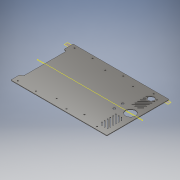
# Autodesk Inventor part: Back
Saved by Autodesk Inventor 2018 (Build 220112000, 112)
## iProperties
Created: 2017-11-12
Part Number: Back
Material: Edelstahl
Document SubType Name: Blech
Density: 8 g/cm^3
Sheet Metal Rule: Standard_mm
Appearance: Halbpoliert
Flat Pattern Width: 22.4 cm
Flat Pattern Length: 34.5 cm
Flat Pattern Area: 772.799 cm^2
Sheet Metal Width: 224,000 mm
Sheet Metal Length: 345,000 mm
Sheet Metal Area: 77279,943 mm^2
Autodesk Inventor part; units mm, degrees
ref_plane "YZ Plane" through (0, 0, 0) normal (1, 0, 0) x (0, 1, 0)
ref_plane "XZ Plane" through (0, 0, 0) normal (0, 1, 0) x (-1, 0, 0)
ref_plane "XY Plane" through (0, 0, 0) normal (0, 0, 1) x (1, 0, 0)
ref_plane "Arbeitsebene1" through (0, 0, 0) normal (0, 0, 1) x (1, 0, 0)
sketch "Skizze1" plane through (0, 0, 0) normal (0, 0, 1) x (1, 0, 0)
  circle A0 centre (70.3399, -192.2557) radius 2.15 construction
  circle A1 centre (-29.6601, -192.2557) radius 2.15 construction
  circle A2 centre (-29.6601, -17.2557) radius 2.15 construction
  circle A3 centre (70.3399, -17.2557) radius 2.15 construction
  arc A4 (-167.6601, 7.2442) -> (-169.6601, 5.2442) centre (-167.6601, 5.2442) ccw construction
  line L0 (-167.6601, 7.2442) -> (173.3399, 7.2442) construction
  arc A5 (175.3399, 5.2442) -> (173.3399, 7.2442) centre (173.3399, 5.2442) ccw construction
  line L1 (175.3399, -214.7557) -> (175.3399, 5.2442) construction
  arc A6 (173.3399, -216.7557) -> (175.3399, -214.7557) centre (173.3399, -214.7557) ccw construction
  line L2 (-167.6601, -216.7557) -> (173.3399, -216.7557) construction
  arc A7 (-169.6601, -214.7557) -> (-167.6601, -216.7557) centre (-167.6601, -214.7557) ccw construction
  line L3 (-169.6601, -188.2557) -> (-169.6601, -214.7557) construction
  arc A8 (-167.6601, -186.2557) -> (-169.6601, -188.2557) centre (-167.6601, -188.2557) ccw construction
  line L4 (105.3399, -186.2557) -> (-167.6601, -186.2557) construction
  arc A9 (105.3399, -186.2557) -> (115.3399, -176.2557) centre (105.3399, -176.2557) ccw construction
  line L5 (115.3399, -33.2557) -> (115.3399, -176.2557) construction
  arc A10 (115.3399, -33.2557) -> (105.3399, -23.2557) centre (105.3399, -33.2557) ccw construction
  line L6 (-167.6601, -23.2557) -> (105.3399, -23.2557) construction
  arc A11 (-169.6601, -21.2557) -> (-167.6601, -23.2557) centre (-167.6601, -21.2557) ccw construction
  line L7 (-169.6601, 5.2442) -> (-169.6601, -21.2557) construction
  line L8 (175.3399, 7.2442) -> (-169.6601, 7.2442)
  line L9 (-169.6601, 7.2442) -> (-169.6601, -216.7557)
  line L10 (-169.6601, -216.7557) -> (175.3399, -216.7557)
  line L11 (175.3399, -216.7557) -> (175.3399, 7.2442)
  circle A12 centre (-29.6601, -17.2557) radius 2.15
  circle A13 centre (-29.6601, -192.2557) radius 2.15
  circle A14 centre (70.3399, -192.2557) radius 2.15
  circle A15 centre (70.3399, -17.2557) radius 2.15
  circle A16 centre (20.3399, -2.7558) radius 2.15
  circle A17 centre (-89.6601, -206.7557) radius 2.15
  circle A18 centre (130.3399, -206.7557) radius 2.15
  circle A19 centre (20.3399, -206.7557) radius 2.15
  circle A20 centre (-89.6601, -2.7558) radius 2.15
  circle A21 centre (130.3399, -2.7558) radius 2.15
  point P0 (0, 0)
  dimension "d0" = 0
  dimension "d1" = 345
  dimension "d2" = 193.4999
  dimension "d3" = 30.4999
  measures "d0" distance between parallel lines of L1 L11
  measures "d1" distance between parallel lines of L1 L9
  measures "d2" distance between parallel lines of L4 L8
  measures "d3" distance between parallel lines of L4 L10
extrude "Grobblech1" add sketch "Skizze1" along normal blind 2 contours L11 L10 L9 L8 | A16 | A17 | A18 | A19 | A20 | A21
fillet "Eckenrundung1" radius 2 4 edges at (-169.6601, -216.7557, 1) (175.3399, -216.7557, 1) (175.3399, 7.2442, 1) (-169.6601, 7.2442, 1)
sketch "Skizze2" plane through (0, 0, 2) normal (0, 0, 1) x (1, 0, 0)
  arc A0 (-167.6601, 7.2442) -> (-169.6601, 5.2442) centre (-167.6601, 5.2442) ccw projected
  line L0 (-169.6601, -214.7557) -> (-169.6601, 5.2442) projected
  arc A1 (-169.6601, -214.7557) -> (-167.6601, -216.7557) centre (-167.6601, -214.7557) ccw projected
  line L1 (173.3399, -216.7557) -> (-167.6601, -216.7557) projected
  arc A2 (173.3399, -216.7557) -> (175.3399, -214.7557) centre (173.3399, -214.7557) ccw projected
  line L2 (175.3399, 5.2442) -> (175.3399, -214.7557) projected
  arc A3 (175.3399, 5.2442) -> (173.3399, 7.2442) centre (173.3399, 5.2442) ccw projected
  line L3 (-167.6601, 7.2442) -> (173.3399, 7.2442) projected
  circle A4 centre (70.3399, -17.2557) radius 2.15 projected
  circle A5 centre (70.3399, -192.2557) radius 2.15 projected
  circle A6 centre (-29.6601, -192.2557) radius 2.15 projected
  circle A7 centre (-29.6601, -17.2557) radius 2.15 projected
  line L4 (-169.6601, -214.7557) -> (-169.6601, 5.2442) projected
  line L5 (-164.6601, -182.7557) -> (-164.6601, -182.7557)
  line L6 (-164.6601, -26.7558) -> (-164.6601, -26.7558)
  line L7 (-159.6601, -31.7558) -> (-159.6601, -177.7557)
  line L8 (-169.6601, -187.7557) -> (-169.6601, -214.7557)
  line L9 (-169.6601, -21.7558) -> (-169.6601, 5.2442)
  arc A8 (-169.6601, -21.7558) -> (-164.6601, -26.7558) centre (-164.6601, -21.7558) ccw
  arc A9 (-159.6601, -31.7558) -> (-164.6601, -26.7558) centre (-164.6601, -31.7558) ccw
  arc A10 (-164.6601, -182.7557) -> (-159.6601, -177.7557) centre (-164.6601, -177.7557) ccw
  arc A11 (-164.6601, -182.7557) -> (-169.6601, -187.7557) centre (-164.6601, -187.7557) ccw
  line L10 (-169.6601, -21.7558) -> (-169.6601, -187.7557)
  point P0 (0, 0)
  point P1 (-169.6601, -182.7557)
  point P2 (-159.6601, -182.7557)
  point P3 (-169.6601, -26.7558)
  point P4 (-159.6601, -26.7558)
  dimension "d6" = 10
  dimension "d7" = 34
  dimension "d8" = 10
  dimension "d9" = 34
  dimension "d10" = 5
  constraints: 12 end point, 10 point on line, 10 tangent, 8 point on circle, 4 centre point, 3 equal radius, 2 collinear, 1 horizontal, 1 perpendicular
  measures "d6" distance of point (-169.66, -182.756) point (-159.66, -182.756)
  measures "d7" distance between parallel lines of L1 L5
  measures "d8" distance of point (-169.66, -26.756) point (-159.66, -26.756)
  measures "d9" distance between parallel lines of L3 L6
  measures "d10" radius of A8
extrude "Extrusion1" cut sketch "Skizze2" against normal through all contours A8 A9 L7 A10 A11 L0
sketch "Skizze3" plane through (0, 0, 2) normal (0, 0, 1) x (1, 0, 0)
  circle A0 centre (148.5119, -104.7557) radius 16.25 projected
  circle A1 centre (148.5119, -104.7557) radius 17.75
  point P0 (0, 0)
  dimension "d27" = 1.5
  constraints: 1 centre point
  measures "d27" radial gap between concentric circles of A0 A1
extrude "Extrusion2" cut sketch "Skizze3" against normal through all contours A0 | A1
sketch "Skizze4" plane through (0, 0, 2) normal (0, 0, 1) x (1, 0, 0)
  line L0 (115.3399, -201.7557) -> (115.3399, -7.7558) construction
  line L1 (244.3399, -104.7557) -> (-238.6601, -104.7557) construction
  circle A0 centre (105.3399, -119.7557) radius 4
  circle A1 centre (105.3399, -89.7557) radius 4
  point P0 (0, 0)
  dimension "d15" = 8
  dimension "d16" = 8
  dimension "d17" = 15
  dimension "d18" = 10
  dimension "d19" = 10
  dimension "d20" = 15
  constraints: 2 centre point, 2 end point, 1 horizontal, 2 other
  measures "d15" diameter of A0
  measures "d16" diameter of A1
  measures "d17" distance from line of L1 A1.centre
  measures "d18" distance from line of L0 A1.centre
  measures "d19" distance from line of L0 A0.centre
  measures "d20" distance from line of L1 A0.centre
extrude "Extrusion3" cut sketch "Skizze4" against normal through all
sketch "Skizze5" plane through (0, 0, 2) normal (0, 0, 1) x (1, 0, 0)
  circle A0 centre (130.3399, -2.7558) radius 2.15 projected
  circle A1 centre (20.3399, -2.7558) radius 2.15 projected
  circle A2 centre (-89.6601, -2.7558) radius 2.15 projected
  circle A3 centre (-89.6601, -206.7557) radius 2.15 projected
  circle A4 centre (20.3399, -206.7557) radius 2.15 projected
  circle A5 centre (130.3399, -206.7557) radius 2.15 projected
  point P0 (0, 0)
extrude "Extrusion4" cut sketch "Skizze5" against normal through all
ref_plane "Arbeitsebene2" through (-167.6601, -104.7557, 0) normal (0, -1, 0) x (1, 0, 0)
sketch "Skizze6" plane through (0, 0, 0) normal (0, 0, -1) x (-1, 0, 0)
  circle A0 centre (154.6601, -2.7558) radius 2.15
  circle A1 centre (154.6601, -206.7557) radius 2.15
  point P0 (0, 0)
  constraints: 2 centre point, 4 other
extrude "Extrusion5" cut sketch "Skizze6" against normal through all
sketch "Skizze7" plane through (0, 0, 0) normal (0, 0, -1) x (-1, 0, 0)
  line L0 (-97.7459, -78.2296) -> (-73.7459, -78.2296) construction
  line L1 (-70.7459, -75.2296) -> (-70.7459, -21.2296) construction
  line L2 (-73.7459, -18.2296) -> (-97.7459, -18.2296) construction
  line L3 (-100.7459, -21.2296) -> (-100.7459, -75.2296) construction
  circle A0 centre (154.6601, -2.7558) radius 2.15 projected
  circle A1 centre (154.6601, -206.7557) radius 2.15 projected
  circle A2 centre (-20.3399, -206.7557) radius 2.15 projected
  circle A3 centre (89.6601, -2.7558) radius 2.15 projected
  circle A4 centre (-130.3399, -2.7558) radius 2.15 projected
  circle A5 centre (-20.3399, -2.7558) radius 2.15 projected
  circle A6 centre (89.6601, -206.7557) radius 2.15 projected
  circle A7 centre (-130.3399, -206.7557) radius 2.15 projected
  circle A8 centre (-105.3399, -119.7557) radius 4 projected
  circle A9 centre (-105.3399, -89.7557) radius 4 projected
  circle A10 centre (-148.5119, -104.7557) radius 17.75 projected
  arc A11 (169.6601, -187.7557) -> (164.6601, -182.7557) centre (164.6601, -187.7557) ccw projected
  arc A12 (159.6601, -177.7557) -> (164.6601, -182.7557) centre (164.6601, -177.7557) ccw projected
  line L4 (159.6601, -177.7557) -> (159.6601, -31.7558) projected
  arc A13 (164.6601, -26.7558) -> (159.6601, -31.7558) centre (164.6601, -31.7558) ccw projected
  arc A14 (164.6601, -26.7558) -> (169.6601, -21.7558) centre (164.6601, -21.7558) ccw projected
  line L5 (169.6601, 5.2442) -> (169.6601, -21.7558) projected
  arc A15 (169.6601, 5.2442) -> (167.6601, 7.2442) centre (167.6601, 5.2442) ccw projected
  line L6 (-173.3399, 7.2442) -> (167.6601, 7.2442) projected
  arc A16 (-173.3399, 7.2442) -> (-175.3399, 5.2442) centre (-173.3399, 5.2442) ccw projected
  line L7 (-175.3399, -214.7557) -> (-175.3399, 5.2442) projected
  arc A17 (-175.3399, -214.7557) -> (-173.3399, -216.7557) centre (-173.3399, -214.7557) ccw projected
  line L8 (167.6601, -216.7557) -> (-173.3399, -216.7557) projected
  arc A18 (167.6601, -216.7557) -> (169.6601, -214.7557) centre (167.6601, -214.7557) ccw projected
  line L9 (169.6601, -187.7557) -> (169.6601, -214.7557) projected
  circle A19 centre (29.6601, -17.2557) radius 2.15 projected
  circle A20 centre (29.6601, -192.2557) radius 2.15 projected
  circle A21 centre (-70.3399, -192.2557) radius 2.15 projected
  circle A22 centre (-70.3399, -17.2557) radius 2.15 projected
  line L10 (-148.5119, -104.7557) -> (-119.1163, -104.7557) construction
  line L11 (-158.66, -131.2539) -> (-120.76, -131.2539) construction
  arc A23 (-156.5439, -143.3701) -> (-154.7761, -145.1378) centre (-155.66, -144.2539) ccw
  arc A24 (-124.7761, -135.1378) -> (-126.5439, -133.3701) centre (-125.66, -134.2539) ccw
  line L12 (-158.66, -131.2539) -> (-122.66, -131.2539) construction
  line L13 (-156.5439, -173.3701) -> (-126.5439, -143.3701)
  line L14 (-155.66, -174.2539) -> (-125.66, -144.2539) construction
  arc A25 (-124.7761, -175.1378) -> (-126.5439, -173.3701) centre (-125.66, -174.2539) ccw
  line L15 (-156.5439, -183.3701) -> (-126.5439, -153.3701)
  line L16 (-155.66, -184.2539) -> (-125.66, -154.2539) construction
  line L17 (-124.7761, -155.1378) -> (-154.7761, -185.1378)
  line L18 (-155.66, -191.2539) -> (-155.66, -137.2539) construction
  line L19 (-125.66, -137.2539) -> (-125.66, -191.2539) construction
  line L20 (-158.66, -197.2539) -> (-158.66, -131.2539) construction
  line L21 (-122.66, -131.2539) -> (-122.66, -197.2539) construction
  arc A26 (-146.5439, -193.3701) -> (-144.7761, -195.1378) centre (-145.66, -194.2539) ccw
  line L22 (-156.5439, -193.3701) -> (-126.5439, -163.3701)
  line L23 (-155.66, -194.2539) -> (-125.66, -164.2539) construction
  line L24 (-124.7761, -165.1378) -> (-154.7761, -195.1378)
  line L25 (-122.66, -197.2539) -> (-158.66, -197.2539) construction
  arc A27 (-156.5439, -163.3701) -> (-154.7761, -165.1378) centre (-155.66, -164.2539) ccw
  line L26 (-146.5439, -193.3701) -> (-126.5439, -173.3701)
  line L27 (-124.7761, -175.1378) -> (-144.7761, -195.1378)
  arc A28 (-156.5439, -153.3701) -> (-154.7761, -155.1378) centre (-155.66, -154.2539) ccw
  line L28 (-124.7761, -185.1378) -> (-134.7761, -195.1378)
  arc A29 (-156.5439, -173.3701) -> (-154.7761, -175.1378) centre (-155.66, -174.2539) ccw
  arc A30 (-124.7761, -185.1378) -> (-126.5439, -183.3701) centre (-125.66, -184.2539) ccw
  arc A31 (-156.5439, -183.3701) -> (-154.7761, -185.1378) centre (-155.66, -184.2539) ccw
  line L29 (-135.66, -194.2539) -> (-125.66, -184.2539) construction
  line L30 (-145.66, -194.2539) -> (-125.66, -174.2539) construction
  arc A32 (-156.5439, -193.3701) -> (-154.7761, -195.1378) centre (-155.66, -194.2539) ccw
  line L31 (-158.66, -197.8539) -> (-120.76, -197.8539) construction
  arc A33 (-124.7761, -145.1378) -> (-126.5439, -143.3701) centre (-125.66, -144.2539) ccw
  arc A34 (-134.7761, -135.1378) -> (-136.5439, -133.3701) centre (-135.66, -134.2539) ccw
  arc A35 (-125.66, -137.2539) -> (-128.66, -134.2539) centre (-128.66, -137.2539) ccw construction
  arc A36 (-144.7761, -135.1378) -> (-146.5439, -133.3701) centre (-145.66, -134.2539) ccw
  arc A37 (-124.7761, -165.1378) -> (-126.5439, -163.3701) centre (-125.66, -164.2539) ccw
  line L32 (-152.66, -134.2539) -> (-128.66, -134.2539) construction
  arc A38 (-152.66, -134.2539) -> (-155.66, -137.2539) centre (-152.66, -137.2539) ccw construction
  line L33 (-144.7761, -135.1378) -> (-154.7761, -145.1378)
  line L34 (-155.66, -144.2539) -> (-145.66, -134.2539) construction
  line L35 (-156.5439, -143.3701) -> (-146.5439, -133.3701)
  line L36 (-134.7761, -135.1378) -> (-154.7761, -155.1378)
  line L37 (-155.66, -154.2539) -> (-135.66, -134.2539) construction
  line L38 (-156.5439, -153.3701) -> (-136.5439, -133.3701)
  line L39 (-156.5439, -163.3701) -> (-126.5439, -133.3701)
  line L40 (-155.66, -164.2539) -> (-125.66, -134.2539) construction
  line L41 (-124.7761, -135.1378) -> (-154.7761, -165.1378)
  line L42 (-124.7761, -145.1378) -> (-154.7761, -175.1378)
  arc A39 (-124.7761, -155.1378) -> (-126.5439, -153.3701) centre (-125.66, -154.2539) ccw
  line L43 (-128.66, -194.2539) -> (-152.66, -194.2539) construction
  arc A40 (-128.66, -194.2539) -> (-125.66, -191.2539) centre (-128.66, -191.2539) ccw construction
  line L44 (-136.5439, -193.3701) -> (-126.5439, -183.3701)
  arc A41 (-155.66, -191.2539) -> (-152.66, -194.2539) centre (-152.66, -191.2539) ccw construction
  arc A42 (-136.5439, -193.3701) -> (-134.7761, -195.1378) centre (-135.66, -194.2539) ccw
  line L45 (-175.3399, -214.7557) -> (-175.3399, 5.2442) projected
  line L46 (-173.3399, -203.5364) -> (-171.4999, -203.5364) construction
  arc A43 (-154.7761, -34.3737) -> (-156.5439, -36.1414) centre (-155.66, -35.2576) ccw
  arc A44 (-154.7761, -44.3737) -> (-156.5439, -46.1414) centre (-155.66, -45.2576) ccw
  arc A45 (-155.66, -72.2576) -> (-152.66, -75.2576) centre (-152.66, -72.2576) ccw construction
  line L47 (-155.66, -65.2576) -> (-145.66, -75.2576) construction
  line L48 (-156.5439, -16.1414) -> (-126.5439, -46.1414)
  arc A46 (-128.66, -75.2576) -> (-125.66, -72.2576) centre (-128.66, -72.2576) ccw construction
  arc A47 (-136.5439, -76.1414) -> (-134.7761, -74.3737) centre (-135.66, -75.2576) ccw
  arc A48 (-154.7761, -54.3737) -> (-156.5439, -56.1414) centre (-155.66, -55.2576) ccw
  line L49 (-158.66, -12.2576) -> (-158.66, -78.2576) construction
  line L50 (-124.7761, -34.3737) -> (-144.7761, -14.3737)
  line L51 (-122.66, -12.2576) -> (-158.66, -12.2576) construction
  arc A49 (-126.5439, -26.1414) -> (-124.7761, -24.3737) centre (-125.66, -25.2576) ccw
  arc A50 (-126.5439, -66.1414) -> (-124.7761, -64.3737) centre (-125.66, -65.2576) ccw
  line L52 (-122.66, -78.2576) -> (-122.66, -12.2576) construction
  arc A51 (-126.5439, -36.1414) -> (-124.7761, -34.3737) centre (-125.66, -35.2576) ccw
  line L53 (-158.66, -78.2576) -> (-120.76, -78.2576) construction
  line L54 (-156.5439, -36.1414) -> (-126.5439, -66.1414)
  arc A52 (-154.7761, -64.3737) -> (-156.5439, -66.1414) centre (-155.66, -65.2576) ccw
  arc A53 (-126.5439, -76.1414) -> (-124.7761, -74.3737) centre (-125.66, -75.2576) ccw
  line L55 (-158.66, -78.2576) -> (-122.66, -78.2576) construction
  arc A54 (-126.5439, -46.1414) -> (-124.7761, -44.3737) centre (-125.66, -45.2576) ccw
  arc A55 (-146.5439, -76.1414) -> (-144.7761, -74.3737) centre (-145.66, -75.2576) ccw
  arc A56 (-125.66, -18.2576) -> (-128.66, -15.2576) centre (-128.66, -18.2576) ccw construction
  line L56 (-124.7761, -44.3737) -> (-154.7761, -14.3737)
  line L57 (-158.66, -11.6576) -> (-120.76, -11.6576) construction
  line L58 (-124.7761, -24.3737) -> (-134.7761, -14.3737)
  line L59 (-144.7761, -74.3737) -> (-154.7761, -64.3737)
  line L60 (-152.66, -75.2576) -> (-128.66, -75.2576) construction
  arc A57 (-134.7761, -14.3737) -> (-136.5439, -16.1414) centre (-135.66, -15.2576) ccw
  line L61 (-136.5439, -16.1414) -> (-126.5439, -26.1414)
  line L62 (-135.66, -15.2576) -> (-125.66, -25.2576) construction
  line L63 (-145.66, -15.2576) -> (-125.66, -35.2576) construction
  arc A58 (-144.7761, -14.3737) -> (-146.5439, -16.1414) centre (-145.66, -15.2576) ccw
  line L64 (-128.66, -15.2576) -> (-152.66, -15.2576) construction
  arc A59 (-152.66, -15.2576) -> (-155.66, -18.2576) centre (-152.66, -18.2576) ccw construction
  arc A60 (-126.5439, -56.1414) -> (-124.7761, -54.3737) centre (-125.66, -55.2576) ccw
  line L65 (-124.7761, -54.3737) -> (-154.7761, -24.3737)
  line L66 (-155.66, -25.2576) -> (-125.66, -55.2576) construction
  line L67 (-156.5439, -26.1414) -> (-126.5439, -56.1414)
  line L68 (-125.66, -72.2576) -> (-125.66, -18.2576) construction
  line L69 (-155.66, -18.2576) -> (-155.66, -72.2576) construction
  line L70 (-124.7761, -64.3737) -> (-154.7761, -34.3737)
  line L71 (-155.66, -35.2576) -> (-125.66, -65.2576) construction
  line L72 (-124.7761, -74.3737) -> (-154.7761, -44.3737)
  line L73 (-155.66, -45.2576) -> (-125.66, -75.2576) construction
  line L74 (-156.5439, -46.1414) -> (-126.5439, -76.1414)
  line L75 (-134.7761, -74.3737) -> (-154.7761, -54.3737)
  line L76 (-155.66, -55.2576) -> (-135.66, -75.2576) construction
  line L77 (-156.5439, -56.1414) -> (-136.5439, -76.1414)
  line L78 (-156.5439, -66.1414) -> (-146.5439, -76.1414)
  line L79 (-146.5439, -16.1414) -> (-126.5439, -36.1414)
  line L80 (-155.66, -15.2576) -> (-125.66, -45.2576) construction
  arc A61 (-154.7761, -14.3737) -> (-156.5439, -16.1414) centre (-155.66, -15.2576) ccw
  arc A62 (-154.7761, -24.3737) -> (-156.5439, -26.1414) centre (-155.66, -25.2576) ccw
  point P0 (0, 0)
  point P1 (-100.7459, -78.2296)
  point P2 (-100.7459, -68.2296)
  point P3 (-100.7459, -58.2296)
  point P4 (-100.7459, -48.2296)
  point P5 (-100.7459, -38.2296)
  point P6 (-100.7459, -28.2296)
  point P7 (-100.7459, -18.2296)
  point P8 (-90.7459, -78.2296)
  point P9 (-80.7459, -78.2296)
  point P10 (-70.7459, -78.2296)
  point P11 (-70.7459, -68.2296)
  point P12 (-70.7459, -58.2296)
  point P13 (-70.7459, -48.2296)
  point P14 (-70.7459, -38.2296)
  point P15 (-70.7459, -28.2296)
  point P16 (-70.7459, -18.2296)
  point P17 (-90.7459, -18.2296)
  point P18 (-80.7459, -18.2296)
  point P19 (-70.7459, -18.2296)
  point P20 (-155.66, -134.2539)
  point P21 (-125.66, -134.2539)
  point P22 (-140.66, -179.2539)
  point P23 (-140.66, -149.2539)
  point P24 (-145.66, -144.2539)
  point P25 (-150.66, -139.2539)
  point P26 (-140.66, -169.2539)
  point P27 (-140.66, -159.2539)
  point P28 (-135.66, -184.2539)
  point P29 (-130.66, -189.2539)
  point P30 (-125.66, -194.2539)
  point P31 (-135.66, -194.2539)
  point P32 (-145.66, -194.2539)
  point P33 (-125.66, -194.2539)
  point P34 (-125.66, -184.2539)
  point P35 (-125.66, -174.2539)
  point P36 (-125.66, -164.2539)
  point P37 (-125.66, -154.2539)
  point P38 (-125.66, -144.2539)
  point P39 (-125.66, -134.2539)
  point P40 (-135.66, -134.2539)
  point P41 (-145.66, -134.2539)
  point P42 (-155.66, -194.2539)
  point P43 (-155.66, -184.2539)
  point P44 (-155.66, -174.2539)
  point P45 (-155.66, -164.2539)
  point P46 (-155.66, -154.2539)
  point P47 (-155.66, -144.2539)
  point P48 (-155.66, -134.2539)
  point P49 (-125.66, -75.2576)
  point P50 (-140.66, -60.2576)
  point P51 (-130.66, -20.2576)
  point P52 (-140.66, -50.2576)
  point P53 (-150.66, -70.2576)
  point P54 (-145.66, -65.2576)
  point P55 (-135.66, -25.2576)
  point P56 (-140.66, -40.2576)
  point P57 (-155.66, -75.2576)
  point P58 (-140.66, -30.2576)
  point P59 (-155.66, -75.2576)
  point P60 (-155.66, -65.2576)
  point P61 (-155.66, -55.2576)
  point P62 (-155.66, -45.2576)
  point P63 (-155.66, -35.2576)
  point P64 (-155.66, -25.2576)
  point P65 (-155.66, -15.2576)
  point P66 (-145.66, -75.2576)
  point P67 (-135.66, -75.2576)
  point P68 (-125.66, -75.2576)
  point P69 (-125.66, -65.2576)
  point P70 (-125.66, -55.2576)
  point P71 (-125.66, -45.2576)
  point P72 (-125.66, -35.2576)
  point P73 (-125.66, -25.2576)
  point P74 (-125.66, -15.2576)
  point P75 (-145.66, -15.2576)
  point P76 (-135.66, -15.2576)
  point P77 (-125.66, -15.2576)
  dimension "d50" = 10
  dimension "d51" = 10
  dimension "d52" = 10
  dimension "d53" = 10
  dimension "d71" = 1.84
  constraints: 180 end point, 98 symmetric about line, 80 point on circle, 40 centre point, 12 point on line, 2 horizontal, 2 vertical, 38 other
  measures "d50" distance of point (-100.746, -78.23) point (-100.746, -68.23)
  measures "d51" distance of point (-100.746, -78.23) point (-90.746, -78.23)
  measures "d52" distance of point (-70.746, -78.23) point (-70.746, -68.23)
  measures "d53" distance of point (-100.746, -18.23) point (-90.746, -18.23)
  measures "d71" distance of L46.start L46.end
extrude "Extrusion7" cut sketch "Skizze7" against normal blind 10 contours L35 A36 L33 A23 | L41 A27 L39 A24 | L13 A33 L42 A29 | L27 A26 L26 A25 | L15 A39 L17 A31 | L22 A37 L24 A32 | L38 A34 L36 A28 | L28 A42 L44 A30 | L70 A50 L54 A43 | L72 A53 L74 A44 | A61 L56 A54 L48 | L77 A48 L75 A47 | A51 L79 A58 L50 | L61 A57 L58 A49 | L59 A55 L78 A52 | L67 A62 L65 A60
sketch "Skizze8" plane through (0, 0, 2) normal (0, 0, 1) x (1, 0, 0)
  arc A0 (124.7761, -64.3737) -> (126.5439, -66.1414) centre (125.66, -65.2576) ccw construction
  line L0 (124.7761, -64.3737) -> (154.7761, -34.3737) construction
  arc A1 (156.5439, -36.1414) -> (154.7761, -34.3737) centre (155.66, -35.2576) ccw construction
  line L1 (156.5439, -36.1414) -> (126.5439, -66.1414) construction
  arc A2 (124.7761, -74.3737) -> (126.5439, -76.1414) centre (125.66, -75.2576) ccw construction
  line L2 (124.7761, -74.3737) -> (154.7761, -44.3737) construction
  arc A3 (156.5439, -46.1414) -> (154.7761, -44.3737) centre (155.66, -45.2576) ccw construction
  line L3 (156.5439, -46.1414) -> (126.5439, -76.1414) construction
  arc A4 (126.5439, -133.3701) -> (124.7761, -135.1378) centre (125.66, -134.2539) ccw projected
  line L4 (126.5439, -133.3701) -> (156.5439, -163.3701) projected
  arc A5 (154.7761, -165.1378) -> (156.5439, -163.3701) centre (155.66, -164.2539) ccw projected
  line L5 (154.7761, -165.1378) -> (124.7761, -135.1378) projected
  arc A6 (126.5439, -153.3701) -> (124.7761, -155.1378) centre (125.66, -154.2539) ccw projected
  line L6 (126.5439, -153.3701) -> (156.5439, -183.3701) projected
  arc A7 (154.7761, -185.1378) -> (156.5439, -183.3701) centre (155.66, -184.2539) ccw projected
  line L7 (154.7761, -185.1378) -> (124.7761, -155.1378) projected
  arc A8 (146.5439, -16.1414) -> (144.7761, -14.3737) centre (145.66, -15.2576) ccw construction
  line L8 (146.5439, -16.1414) -> (126.5439, -36.1414) construction
  arc A9 (124.7761, -34.3737) -> (126.5439, -36.1414) centre (125.66, -35.2576) ccw construction
  line L9 (124.7761, -34.3737) -> (144.7761, -14.3737) construction
  arc A10 (136.5439, -133.3701) -> (134.7761, -135.1378) centre (135.66, -134.2539) ccw projected
  line L10 (136.5439, -133.3701) -> (156.5439, -153.3701) projected
  arc A11 (154.7761, -155.1378) -> (156.5439, -153.3701) centre (155.66, -154.2539) ccw projected
  line L11 (154.7761, -155.1378) -> (134.7761, -135.1378) projected
  arc A12 (124.7761, -24.3737) -> (126.5439, -26.1414) centre (125.66, -25.2576) ccw construction
  line L12 (124.7761, -24.3737) -> (134.7761, -14.3737) construction
  arc A13 (136.5439, -16.1414) -> (134.7761, -14.3737) centre (135.66, -15.2576) ccw construction
  line L13 (136.5439, -16.1414) -> (126.5439, -26.1414) construction
  arc A14 (134.7761, -195.1378) -> (136.5439, -193.3701) centre (135.66, -194.2539) ccw projected
  line L14 (134.7761, -195.1378) -> (124.7761, -185.1378) projected
  arc A15 (126.5439, -183.3701) -> (124.7761, -185.1378) centre (125.66, -184.2539) ccw projected
  line L15 (126.5439, -183.3701) -> (136.5439, -193.3701) projected
  arc A16 (146.5439, -133.3701) -> (144.7761, -135.1378) centre (145.66, -134.2539) ccw projected
  line L16 (146.5439, -133.3701) -> (156.5439, -143.3701) projected
  arc A17 (154.7761, -145.1378) -> (156.5439, -143.3701) centre (155.66, -144.2539) ccw projected
  line L17 (154.7761, -145.1378) -> (144.7761, -135.1378) projected
  arc A18 (156.5439, -66.1414) -> (154.7761, -64.3737) centre (155.66, -65.2576) ccw construction
  line L18 (156.5439, -66.1414) -> (146.5439, -76.1414) construction
  arc A19 (144.7761, -74.3737) -> (146.5439, -76.1414) centre (145.66, -75.2576) ccw construction
  line L19 (144.7761, -74.3737) -> (154.7761, -64.3737) construction
  arc A20 (126.5439, -173.3701) -> (124.7761, -175.1378) centre (125.66, -174.2539) ccw projected
  line L20 (126.5439, -173.3701) -> (146.5439, -193.3701) projected
  arc A21 (144.7761, -195.1378) -> (146.5439, -193.3701) centre (145.66, -194.2539) ccw projected
  line L21 (144.7761, -195.1378) -> (124.7761, -175.1378) projected
  arc A22 (156.5439, -56.1414) -> (154.7761, -54.3737) centre (155.66, -55.2576) ccw construction
  line L22 (156.5439, -56.1414) -> (136.5439, -76.1414) construction
  arc A23 (134.7761, -74.3737) -> (136.5439, -76.1414) centre (135.66, -75.2576) ccw construction
  line L23 (134.7761, -74.3737) -> (154.7761, -54.3737) construction
  arc A24 (154.7761, -195.1378) -> (156.5439, -193.3701) centre (155.66, -194.2539) ccw projected
  line L24 (154.7761, -195.1378) -> (124.7761, -165.1378) projected
  arc A25 (126.5439, -163.3701) -> (124.7761, -165.1378) centre (125.66, -164.2539) ccw projected
  line L25 (126.5439, -163.3701) -> (156.5439, -193.3701) projected
  arc A26 (126.5439, -143.3701) -> (124.7761, -145.1378) centre (125.66, -144.2539) ccw projected
  line L26 (126.5439, -143.3701) -> (156.5439, -173.3701) projected
  arc A27 (154.7761, -175.1378) -> (156.5439, -173.3701) centre (155.66, -174.2539) ccw projected
  line L27 (154.7761, -175.1378) -> (124.7761, -145.1378) projected
  arc A28 (156.5439, -26.1414) -> (154.7761, -24.3737) centre (155.66, -25.2576) ccw construction
  line L28 (156.5439, -26.1414) -> (126.5439, -56.1414) construction
  arc A29 (124.7761, -54.3737) -> (126.5439, -56.1414) centre (125.66, -55.2576) ccw construction
  line L29 (124.7761, -54.3737) -> (154.7761, -24.3737) construction
  arc A30 (124.7761, -44.3737) -> (126.5439, -46.1414) centre (125.66, -45.2576) ccw construction
  line L30 (124.7761, -44.3737) -> (154.7761, -14.3737) construction
  arc A31 (156.5439, -16.1414) -> (154.7761, -14.3737) centre (155.66, -15.2576) ccw construction
  line L31 (156.5439, -16.1414) -> (126.5439, -46.1414) construction
  circle A32 centre (-154.6601, -2.7558) radius 2.15 projected
  circle A33 centre (-154.6601, -206.7557) radius 2.15 projected
  circle A34 centre (20.3399, -206.7557) radius 2.15 projected
  circle A35 centre (-89.6601, -2.7558) radius 2.15 projected
  circle A36 centre (130.3399, -2.7558) radius 2.15 projected
  circle A37 centre (20.3399, -2.7558) radius 2.15 projected
  circle A38 centre (-89.6601, -206.7557) radius 2.15 projected
  circle A39 centre (130.3399, -206.7557) radius 2.15 projected
  circle A40 centre (105.3399, -119.7557) radius 4 projected
  circle A41 centre (105.3399, -89.7557) radius 4 projected
  circle A42 centre (148.5119, -104.7557) radius 17.75 projected
  arc A43 (-164.6601, -182.7557) -> (-169.6601, -187.7557) centre (-164.6601, -187.7557) ccw projected
  line L32 (-169.6601, -214.7557) -> (-169.6601, -187.7557) projected
  arc A44 (-169.6601, -214.7557) -> (-167.6601, -216.7557) centre (-167.6601, -214.7557) ccw projected
  line L33 (173.3399, -216.7557) -> (-167.6601, -216.7557) projected
  arc A45 (173.3399, -216.7557) -> (175.3399, -214.7557) centre (173.3399, -214.7557) ccw projected
  line L34 (175.3399, 5.2442) -> (175.3399, -214.7557) projected
  arc A46 (175.3399, 5.2442) -> (173.3399, 7.2442) centre (173.3399, 5.2442) ccw projected
  line L35 (-167.6601, 7.2442) -> (173.3399, 7.2442) projected
  arc A47 (-167.6601, 7.2442) -> (-169.6601, 5.2442) centre (-167.6601, 5.2442) ccw projected
  line L36 (-169.6601, -21.7558) -> (-169.6601, 5.2442) projected
  arc A48 (-169.6601, -21.7558) -> (-164.6601, -26.7558) centre (-164.6601, -21.7558) ccw projected
  arc A49 (-159.6601, -31.7558) -> (-164.6601, -26.7558) centre (-164.6601, -31.7558) ccw projected
  line L37 (-159.6601, -31.7558) -> (-159.6601, -177.7557) projected
  arc A50 (-164.6601, -182.7557) -> (-159.6601, -177.7557) centre (-164.6601, -177.7557) ccw projected
  circle A51 centre (70.3399, -17.2557) radius 2.15 projected
  circle A52 centre (70.3399, -192.2557) radius 2.15 projected
  circle A53 centre (-29.6601, -192.2557) radius 2.15 projected
  circle A54 centre (-29.6601, -17.2557) radius 2.15 projected
  line L38 (155.66, -15.2576) -> (125.66, -15.2576) construction
  line L39 (125.66, -15.2576) -> (125.66, -75.2576) construction
  line L40 (125.66, -75.2576) -> (155.66, -75.2576) construction
  line L41 (155.66, -75.2576) -> (155.66, -15.2576) construction
  line L42 (155.66, -15.2576) -> (125.66, -75.2576) construction
  line L43 (125.66, -15.2576) -> (155.66, -75.2576) construction
  circle A55 centre (140.66, -22.7558) radius 13.75
  circle A56 centre (130.3399, -2.7558) radius 3.75 construction
  point P0 (0, 0)
  dimension "d75" = 27.5
  dimension "d76" = 34.6799
  dimension "d77" = 30
  dimension "d83" = 7.5
  constraints: 12 end point, 2 centre point, 2 parallel, 1 coincident, 1 horizontal, 1 perpendicular
  measures "d75" diameter of A55
  measures "d76" distance from line of L34 A55.centre
  measures "d77" distance from line of L35 A55.centre
  measures "d83" diameter of A56
extrude "Extrusion8" add sketch "Skizze8" against normal blind 2 contours A55
sketch "Skizze9" plane through (0, 0, 2) normal (0, 0, 1) x (1, 0, 0)
  line L0 (156.5439, -46.1414) -> (126.5439, -76.1414) projected
  arc A0 (124.7761, -74.3737) -> (126.5439, -76.1414) centre (125.66, -75.2576) ccw projected
  line L1 (124.7761, -74.3737) -> (154.7761, -44.3737) projected
  arc A1 (126.9201, -22.2297) -> (127.1864, -25.4989) centre (140.66, -22.7558) ccw construction
  line L2 (156.5439, -36.1414) -> (126.5439, -66.1414) projected
  arc A2 (124.7761, -64.3737) -> (126.5439, -66.1414) centre (125.66, -65.2576) ccw projected
  line L3 (124.7761, -64.3737) -> (154.7761, -34.3737) projected
  arc A3 (129.0411, -30.1087) -> (130.5789, -32.1064) centre (140.66, -22.7558) ccw projected
  line L4 (148.9898, -33.6955) -> (126.5439, -56.1414) projected
  arc A4 (124.7761, -54.3737) -> (126.5439, -56.1414) centre (125.66, -55.2576) ccw projected
  line L5 (124.7761, -54.3737) -> (142.8137, -36.3361) projected
  arc A5 (142.8137, -36.3361) -> (148.9898, -33.6955) centre (140.66, -22.7558) ccw projected
  line L6 (136.7478, -35.9375) -> (126.5439, -46.1414) projected
  arc A6 (124.7761, -44.3737) -> (126.5439, -46.1414) centre (125.66, -45.2576) ccw projected
  line L7 (124.7761, -44.3737) -> (134.2366, -34.9132) projected
  arc A7 (134.2366, -34.9132) -> (136.7478, -35.9375) centre (140.66, -22.7558) ccw projected
  arc A8 (156.5439, -46.1414) -> (154.7761, -44.3737) centre (155.66, -45.2576) ccw projected
  arc A9 (156.5439, -36.1414) -> (154.7761, -34.3737) centre (155.66, -35.2576) ccw projected
  arc A10 (151.5997, -31.0856) -> (154.2403, -24.9095) centre (140.66, -22.7558) ccw projected
  line L8 (154.2403, -24.9095) -> (154.7761, -24.3737) projected
  arc A11 (156.5439, -26.1414) -> (154.7761, -24.3737) centre (155.66, -25.2576) ccw projected
  line L9 (156.5439, -26.1414) -> (151.5997, -31.0856) projected
  arc A12 (153.8417, -18.8436) -> (152.8174, -16.3324) centre (140.66, -22.7558) ccw projected
  line L10 (152.8174, -16.3324) -> (154.7761, -14.3737) projected
  arc A13 (156.5439, -16.1414) -> (154.7761, -14.3737) centre (155.66, -15.2576) ccw projected
  line L11 (156.5439, -16.1414) -> (153.8417, -18.8436) projected
  arc A14 (126.5439, -133.3701) -> (124.7761, -135.1378) centre (125.66, -134.2539) ccw projected
  line L12 (126.5439, -133.3701) -> (156.5439, -163.3701) projected
  arc A15 (154.7761, -165.1378) -> (156.5439, -163.3701) centre (155.66, -164.2539) ccw projected
  line L13 (154.7761, -165.1378) -> (124.7761, -135.1378) projected
  arc A16 (126.5439, -153.3701) -> (124.7761, -155.1378) centre (125.66, -154.2539) ccw projected
  line L14 (126.5439, -153.3701) -> (156.5439, -183.3701) projected
  arc A17 (154.7761, -185.1378) -> (156.5439, -183.3701) centre (155.66, -184.2539) ccw projected
  line L15 (154.7761, -185.1378) -> (124.7761, -155.1378) projected
  line L16 (130.5789, -32.1064) -> (126.5439, -36.1414) projected
  arc A18 (124.7761, -34.3737) -> (126.5439, -36.1414) centre (125.66, -35.2576) ccw projected
  line L17 (124.7761, -34.3737) -> (129.0411, -30.1087) projected
  arc A19 (136.5439, -133.3701) -> (134.7761, -135.1378) centre (135.66, -134.2539) ccw projected
  line L18 (136.5439, -133.3701) -> (156.5439, -153.3701) projected
  arc A20 (154.7761, -155.1378) -> (156.5439, -153.3701) centre (155.66, -154.2539) ccw projected
  line L19 (154.7761, -155.1378) -> (134.7761, -135.1378) projected
  arc A21 (124.7761, -24.3737) -> (126.5439, -26.1414) centre (125.66, -25.2576) ccw construction
  line L20 (124.7761, -24.3737) -> (126.9201, -22.2297) projected
  line L21 (127.1864, -25.4989) -> (126.5439, -26.1414) construction
  arc A22 (134.7761, -195.1378) -> (136.5439, -193.3701) centre (135.66, -194.2539) ccw projected
  line L22 (134.7761, -195.1378) -> (124.7761, -185.1378) projected
  arc A23 (126.5439, -183.3701) -> (124.7761, -185.1378) centre (125.66, -184.2539) ccw projected
  line L23 (126.5439, -183.3701) -> (136.5439, -193.3701) projected
  arc A24 (146.5439, -133.3701) -> (144.7761, -135.1378) centre (145.66, -134.2539) ccw projected
  line L24 (146.5439, -133.3701) -> (156.5439, -143.3701) projected
  arc A25 (154.7761, -145.1378) -> (156.5439, -143.3701) centre (155.66, -144.2539) ccw projected
  line L25 (154.7761, -145.1378) -> (144.7761, -135.1378) projected
  arc A26 (156.5439, -66.1414) -> (154.7761, -64.3737) centre (155.66, -65.2576) ccw projected
  line L26 (156.5439, -66.1414) -> (146.5439, -76.1414) projected
  arc A27 (144.7761, -74.3737) -> (146.5439, -76.1414) centre (145.66, -75.2576) ccw projected
  line L27 (144.7761, -74.3737) -> (154.7761, -64.3737) projected
  arc A28 (126.5439, -173.3701) -> (124.7761, -175.1378) centre (125.66, -174.2539) ccw projected
  line L28 (126.5439, -173.3701) -> (146.5439, -193.3701) projected
  arc A29 (144.7761, -195.1378) -> (146.5439, -193.3701) centre (145.66, -194.2539) ccw projected
  line L29 (144.7761, -195.1378) -> (124.7761, -175.1378) projected
  arc A30 (156.5439, -56.1414) -> (154.7761, -54.3737) centre (155.66, -55.2576) ccw projected
  line L30 (156.5439, -56.1414) -> (136.5439, -76.1414) projected
  arc A31 (134.7761, -74.3737) -> (136.5439, -76.1414) centre (135.66, -75.2576) ccw projected
  line L31 (134.7761, -74.3737) -> (154.7761, -54.3737) projected
  arc A32 (154.7761, -195.1378) -> (156.5439, -193.3701) centre (155.66, -194.2539) ccw projected
  line L32 (154.7761, -195.1378) -> (124.7761, -165.1378) projected
  arc A33 (126.5439, -163.3701) -> (124.7761, -165.1378) centre (125.66, -164.2539) ccw projected
  line L33 (126.5439, -163.3701) -> (156.5439, -193.3701) projected
  arc A34 (126.5439, -143.3701) -> (124.7761, -145.1378) centre (125.66, -144.2539) ccw projected
  line L34 (126.5439, -143.3701) -> (156.5439, -173.3701) projected
  arc A35 (154.7761, -175.1378) -> (156.5439, -173.3701) centre (155.66, -174.2539) ccw projected
  line L35 (154.7761, -175.1378) -> (124.7761, -145.1378) projected
  circle A36 centre (-154.6601, -2.7558) radius 2.15 projected
  circle A37 centre (-154.6601, -206.7557) radius 2.15 projected
  circle A38 centre (20.3399, -206.7557) radius 2.15 projected
  circle A39 centre (-89.6601, -2.7558) radius 2.15 projected
  circle A40 centre (130.3399, -2.7558) radius 2.15 projected
  circle A41 centre (20.3399, -2.7558) radius 2.15 projected
  circle A42 centre (-89.6601, -206.7557) radius 2.15 projected
  circle A43 centre (130.3399, -206.7557) radius 2.15 projected
  circle A44 centre (105.3399, -119.7557) radius 4 projected
  circle A45 centre (105.3399, -89.7557) radius 4 projected
  circle A46 centre (148.5119, -104.7557) radius 17.75 projected
  arc A47 (-164.6601, -182.7557) -> (-169.6601, -187.7557) centre (-164.6601, -187.7557) ccw projected
  line L36 (-169.6601, -214.7557) -> (-169.6601, -187.7557) projected
  arc A48 (-169.6601, -214.7557) -> (-167.6601, -216.7557) centre (-167.6601, -214.7557) ccw projected
  line L37 (173.3399, -216.7557) -> (-167.6601, -216.7557) projected
  arc A49 (173.3399, -216.7557) -> (175.3399, -214.7557) centre (173.3399, -214.7557) ccw projected
  line L38 (175.3399, 5.2442) -> (175.3399, -214.7557) projected
  arc A50 (175.3399, 5.2442) -> (173.3399, 7.2442) centre (173.3399, 5.2442) ccw projected
  line L39 (-167.6601, 7.2442) -> (173.3399, 7.2442) projected
  arc A51 (-167.6601, 7.2442) -> (-169.6601, 5.2442) centre (-167.6601, 5.2442) ccw projected
  line L40 (-169.6601, -21.7558) -> (-169.6601, 5.2442) projected
  arc A52 (-169.6601, -21.7558) -> (-164.6601, -26.7558) centre (-164.6601, -21.7558) ccw projected
  arc A53 (-159.6601, -31.7558) -> (-164.6601, -26.7558) centre (-164.6601, -31.7558) ccw projected
  line L41 (-159.6601, -31.7558) -> (-159.6601, -177.7557) projected
  arc A54 (-164.6601, -182.7557) -> (-159.6601, -177.7557) centre (-164.6601, -177.7557) ccw projected
  circle A55 centre (70.3399, -17.2557) radius 2.15 projected
  circle A56 centre (70.3399, -192.2557) radius 2.15 projected
  circle A57 centre (-29.6601, -192.2557) radius 2.15 projected
  circle A58 centre (-29.6601, -17.2557) radius 2.15 projected
  arc A59 (129.91, -22.7753) -> (130.9, -18.2498) centre (140.66, -22.7558) ccw
  line L42 (124.7761, -24.3737) -> (126.9201, -22.2297) projected
  line L43 (126.9837, -25.7016) -> (129.91, -22.7753)
  line L44 (125.0628, -24.087) -> (130.9, -18.2498)
  line L45 (127.1864, -25.4989) -> (126.5439, -26.1414) construction
  line L46 (125.0628, -24.087) -> (126.9837, -25.7016)
  point P0 (0, 0)
  dimension "d80" = 21.5
  dimension "d85" = 130.046
  dimension "d86" = 54.8023
  constraints: 6 end point, 2 collinear, 2 point on circle, 2 point on line, 1 centre point, 1 coincident
  measures "d80" diameter of A59
  measures "d85" angle of L38 L46
  measures "d86" distance from line of L38.start L46
extrude "Extrusion10" cut sketch "Skizze9" against normal blind 2 contours L20 L44 A59 L43 L46
equation "\"d8\" = d6"
equation "\"d9\" = d7"
equation "\"d19\" = d18"
equation "\"d20\" = d17"
equation "\"d4\" = Stärke"
equation "\"Biegeradius\" = Stärke"
equation "\"BreiteBiegungsfreistellung\" = Stärke"
equation "\"TiefeBiegungsfreistellung\" = 0.5 * Stärke"
equation "\"GrößeEckenfreistellung\" = 4 * Stärke"
equation "\"MinimalRest\" = 2 * Stärke"
equation "\"Übergangsradius\" = Biegeradius"
equation "\"JacobiRadiusGröße\" = Biegeradius"
equation "\"Abstandsgröße\" = Stärke"
equation "\"Stärke\" = 2"
